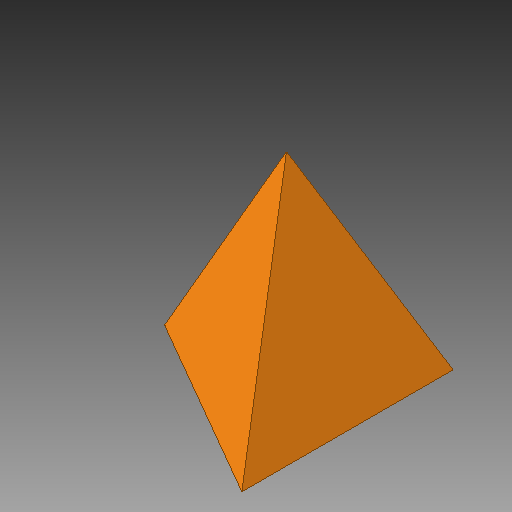
# Autodesk Inventor part: marker pyramid
Saved by Autodesk Inventor 2019 (Build 230136000, 136)
## iProperties
Created: 2018-10-11
Part Number: marker pyramid
Material: ABS Plastic
Document SubType Name: Modeling
Designer: User
Density: 1.06 g/cm^3
Appearance: Orange
Author: User
Autodesk Inventor part; units mm, degrees
ref_plane "YZ Plane" through (0, 0, 0) normal (1, 0, 0) x (0, 1, 0)
ref_plane "XY Plane" through (0, 0, 0) normal (0, 0, 1) x (1, 0, 0)
sketch "Sketch1" plane through (0, 0, 0) normal (0, 1, 0) x (-1, 0, 0)
  line L0 (0, 0) -> (87.9856, -50.8)
  line L1 (87.9856, -50.8) -> (0, -101.6)
  line L2 (0, -101.6) -> (0, 0)
  dimension "d0" = 50.8
  dimension "d1" = 101.6
  dimension "d2" = 87.9856
  constraints: 6 end point, 1 vertical
  measures "d0" vertical distance of L1.end L0.end
  measures "d1" distance of L1.end L0.start
  measures "d2" distance from line of L0.end L2
ref_plane "Work Plane1" through (0, 101.6, 0) normal (0, 1, 0) x (-1, 0, 0)
sketch "Sketch2" plane through (0, 101.6, 0) normal (0, 1, 0) x (-1, 0, 0)
  line L0 (87.9856, -50.8) -> (0, -101.6) projected
  line L1 (0, 0) -> (87.9856, -50.8) projected
  line L2 (0, -101.6) -> (0, 0) projected
  line L3 (43.9928, -76.2) -> (29.3318, -50.7952)
  line L4 (29.3318, -50.7952) -> (43.3864, -25.0499)
  line L5 (29.3318, -50.7952) -> (0, -50.7952)
  constraints: 6 end point, 2 equal length, 2 point on line, 1 midpoint, 1 perpendicular
loft "Loft1" add profiles "Sketch1" section 2 point at (-29.3318, 101.6, -50.7952)
sketch "Sketch3" plane through (0, 0, -101.6) normal (0, -1, 0) x (1, 0, 0)
  line L0 (-29.3421, 50.7772) -> (-43.9928, 76.2)
  line L1 (0, 101.6) -> (-87.9856, 50.8) projected
  line L2 (-29.3421, 50.7772) -> (0, 50.7772)
  line L3 (0, 0) -> (0, 101.6) projected
  line L4 (-29.3421, 50.7772) -> (-42.6757, 24.6396)
  line L5 (-87.9856, 50.8) -> (0, 0) projected
  constraints: 6 end point, 2 equal length, 2 point on line, 1 horizontal, 1 midpoint
hole "Hole1" at (-29.3421, 0, -50.8228) direction (0, 1, 0) diameter 7.62 depth 50.8
equation "\"d0\" = 0.5 * d1"
body "Solid1"
